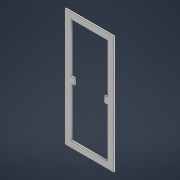
# Autodesk Inventor part: Shoulder_Cube_TestFit_V1
Saved by Autodesk Inventor 2022 (Build 260153000, 153)
## iProperties
Created: 2023-05-16
Part Number: Shoulder_Cube_TestFit_V1
Material: Generic
Document SubType Name: Modeling
Designer: Karl Spiteri
Density: 1 g/cm^3
Appearance: Default
Author: Karl Spiteri
Autodesk Inventor part; units mm, degrees
ref_plane "YZ Plane" through (0, 0, 0) normal (1, 0, 0) x (0, 1, 0)
ref_plane "XZ Plane" through (0, 0, 0) normal (0, 1, 0) x (-1, 0, 0)
ref_plane "XY Plane" through (0, 0, 0) normal (0, 0, 1) x (1, 0, 0)
sketch "Sketch1" plane through (0, 0, 0) normal (0, 0, 1) x (1, 0, 0)
  line L0 (0, 0) -> (-75, 0)
  line L1 (-75, 0) -> (-75, 180)
  line L2 (-75, 180) -> (0, 180)
  line L3 (0, 180) -> (0, 0)
  line L4 (-65, 170) -> (-10, 170)
  line L5 (-10, 10) -> (-65, 10)
  line L6 (-60, 85) -> (-65, 85)
  line L7 (-65, 95) -> (-60, 95)
  line L8 (-60, 95) -> (-60, 85)
  line L9 (-10, 85) -> (-15, 85)
  line L10 (-15, 85) -> (-15, 95)
  line L11 (-15, 95) -> (-10, 95)
  line L12 (-65, 10) -> (-65, 85)
  line L13 (-65, 95) -> (-65, 170)
  line L14 (-10, 170) -> (-10, 95)
  line L15 (-10, 85) -> (-10, 10)
  dimension "d35" = 75
  dimension "d36" = 180
  dimension "d37" = 55
  dimension "d38" = 160
  dimension "d44" = 5
  dimension "d45" = 10
  dimension "d46" = 5
  dimension "d47" = 10
  constraints: 32 end point, 5 parallel, 4 horizontal, 4 perpendicular
  measures "d35" distance of L1.end L2.end
  measures "d36" distance of L0.end L1.end
  measures "d37" distance of L5.start L5.end
  measures "d38" distance of L4.end L5.start
  measures "d44" distance of L7.start L7.end
  measures "d45" distance of L6.end L7.start
  measures "d46" distance of L10.end L11.end
  measures "d47" distance of L9.end L10.end
extrude "Extrusion6" add sketch "Sketch1" along normal blind 2
body "Solid4"
